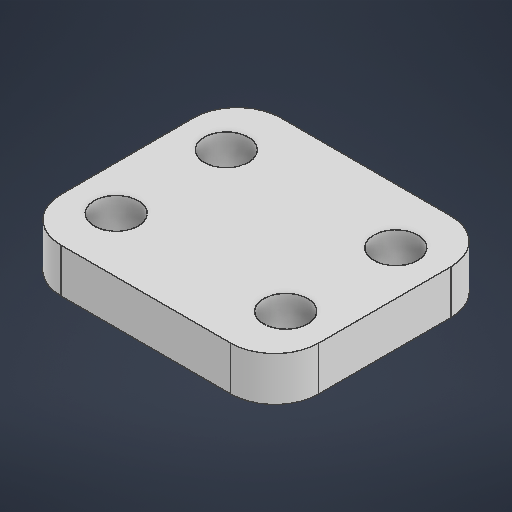
# Autodesk Inventor part: rigid_support3
Saved by Autodesk Inventor 2026.1 (Build 301233000, 233)
## iProperties
Created: 2025-10-28
Part Number: rigid_support3
Material: Generic
Document SubType Name: Modeling
Designer: emanuel
Density: 1 g/cm^3
Appearance: Default
Author: emanuel
Autodesk Inventor part; units mm, degrees
ref_plane "YZ Plane" through (0, 0, 0) normal (1, 0, 0) x (0, 1, 0)
ref_plane "XZ Plane" through (0, 0, 0) normal (0, 1, 0) x (-1, 0, 0)
ref_plane "XY Plane" through (0, 0, 0) normal (0, 0, 1) x (1, 0, 0)
sketch "Sketch1" plane through (0, 0, 0) normal (0, 1, 0) x (-1, 0, 0)
  line L0 (0, 0) -> (8, 0)
  line L1 (8, 0) -> (8, -20)
  line L2 (8, -20) -> (0, -20)
  line L3 (0, -20) -> (0, 0)
  line L4 (0, 0) -> (-3.7, 0)
  line L5 (-3.7, 0) -> (-3.7, -20)
  line L6 (-3.7, -20) -> (0, -20)
  line L7 (0, -20) -> (0, 0)
  line L8 (8, 0) -> (4, 0)
  line L9 (4, 0) -> (4, -5)
  line L10 (4, -5) -> (8, -5)
  line L11 (8, -5) -> (8, 0)
  line L12 (4, -5) -> (4, -15)
  circle A0 centre (4, -5) radius 2
  circle A1 centre (4, -15) radius 2
  line L13 (-7.4, 0) -> (-15.4, 0)
  line L14 (-15.4, 0) -> (-15.4, -20)
  line L15 (-15.4, -20) -> (-7.4, -20)
  line L16 (-7.4, -20) -> (-7.4, 0)
  line L17 (-7.4, 0) -> (-3.7, 0)
  line L18 (-3.7, -20) -> (-7.4, -20)
  line L19 (-7.4, -20) -> (-7.4, 0)
  line L20 (-15.4, 0) -> (-11.4, 0)
  line L21 (-11.4, 0) -> (-11.4, -5)
  line L22 (-11.4, -5) -> (-15.4, -5)
  line L23 (-15.4, -5) -> (-15.4, 0)
  line L24 (-11.4, -5) -> (-11.4, -15)
  circle A2 centre (-11.4, -5) radius 2
  circle A3 centre (-11.4, -15) radius 2
  dimension "d0" = 8
  dimension "d1" = 20
  dimension "d2" = 3.7
  dimension "d3" = 4
  dimension "d4" = 5
  dimension "d5" = 10
  dimension "d6" = 4
  dimension "d7" = 4
  constraints: 50 end point, 11 symmetric about line, 6 parallel, 4 centre point, 4 coincident, 3 horizontal, 3 perpendicular, 2 point on line, 1 vertical, 2 other
  measures "d0" distance of L1.end L2.end
  measures "d1" distance of L0.end L1.end
  measures "d2" distance of L6.end L5.end
  measures "d3" distance of L10.end L9.end
  measures "d4" distance of L9.end L8.end
  measures "d5" distance of L9.end L12.end
  measures "d6" diameter of A0
  measures "d7" diameter of A1
extrude "Extrusion1" add sketch "Sketch1" along normal blind 4 contours L0 L9 A0 L10 L1 L2 L3 | L3 L6 L5 L4 | L0 L1 L10 A0 L9 | L5 L18 L16 L17 | L16 L15 L14 L22 A2 L21 L13 | L21 A2 L22 L14 L13
fillet "Fillet1" radius 4 4 edges at (-8, 2, 0) (15.4, 2, 0) (15.4, 2, -20) (-8, 2, -20)
body "Solid1"
